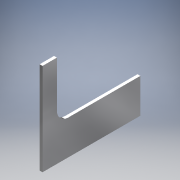
# Autodesk Inventor part: Front Brace 2
Saved by Autodesk Inventor 2019.4 (Build 234330000, 330)
## iProperties
Created: 2020-01-06
Part Number: Front Brace 2
Material: Aluminum 6061
Document SubType Name: Modeling
Designer: Mark
Mass: 171.45 g
Surface Area: 287 cm^2
Volume: 63.5 cm^3
Density: 2.7 g/cm^3
Appearance: Aluminum - Flat
Author: Mark
Autodesk Inventor part; units mm, degrees
ref_plane "YZ Plane" through (0, 0, 0) normal (1, 0, 0) x (0, 1, 0)
ref_plane "XZ Plane" through (0, 0, 0) normal (0, 1, 0) x (-1, 0, 0)
ref_plane "XY Plane" through (0, 0, 0) normal (0, 0, 1) x (1, 0, 0)
sketch "Sketch1" plane through (0, 0, 0) normal (1, 0, 0) x (0, 1, 0)
  line L0 (0, 0) -> (160, 0)
  line L1 (160, 0) -> (160, -25)
  line L2 (160, -25) -> (0, -25)
  line L3 (0, -25) -> (0, 0)
  line L4 (0, -25) -> (60, -25)
  line L5 (60, -25) -> (60, -145)
  line L6 (60, -145) -> (0, -145)
  line L7 (0, -145) -> (0, -25)
  dimension "d0" = 160
  dimension "d1" = 25
  dimension "d2" = 60
  dimension "d3" = 120
  constraints: 16 end point, 4 parallel, 2 horizontal, 2 perpendicular
  measures "d0" distance of L1.end L2.end
  measures "d1" distance of L0.end L1.end
  measures "d2" distance of L5.end L6.end
  measures "d3" distance of L4.end L5.end
extrude "Extrusion1" add sketch "Sketch1" along normal blind 5
fillet "Fillet1" radius 20 1 edges at (2.5, 60, -25)
body "Solid1"
